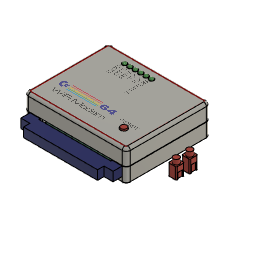
C64-WiFi_UP_PCB2 v9 (Autodesk Fusion 360 design; units mm, degrees)
Autodesk Fusion 360 part; units mm, degrees
note: some values were not read from the file. Set by a fixed rule: which sketch regions a step uses.
(part 1 of 3)
sketch "dxf_import" plane through (0, 0, 0) normal (0, 0, 1) x (1, 0, 0) in component "PCB"
  arc A0 (1, 59) -> (0, 58.08) centre (0.96, 58.04) ccw
  arc A1 (52.3, 0) -> (53.3, 1) centre (52.3, 1) ccw
  arc A2 (53.3, 58.08) -> (52.3, 59) centre (52.34, 58.04) ccw
  circle A3 centre (49.3, 54.7) radius 1.651
  circle A4 centre (4, 12.8) radius 1.651
  line L0 (1, 0) -> (52.3, 0)
  arc A5 (0, 1) -> (1, 0) centre (1, 1) ccw
  arc A6 (48.0347, 39.7544) -> (48.935, 40.0818) centre (48.0347, 41.156) ccw
  line L1 (17.0663, 30.1863) -> (17.0663, 28.2813)
  line L2 (18.6538, 30.8362) -> (19.9238, 31.4713)
  line L3 (21.5113, 30.1863) -> (17.0663, 30.1863)
  line L4 (18.6538, 32.1063) -> (18.6538, 30.8362)
  line L5 (21.543, 34.5271) -> (21.543, 32.6729)
  line L6 (34.0519, 18.9119) -> (34.0519, 17.9594)
  line L7 (33.7344, 18.4944) -> (34.0519, 18.9119)
  line L8 (33.2582, 18.4944) -> (33.2582, 16.2717)
  line L9 (33.0407, 18.9118) -> (33.2582, 18.4944)
  line L10 (21.543, 26.1804) -> (17.987, 26.1804)
  line L11 (33.7345, 16.2718) -> (34.0519, 15.9544)
  line L12 (21.5113, 28.2813) -> (21.5113, 30.1863)
  line L13 (34.0519, 18.9119) -> (32.7819, 18.9119)
  line L14 (17.987, 28.0346) -> (21.543, 28.0346)
  line L15 (17.0663, 32.4237) -> (17.0663, 30.5188)
  line L16 (21.543, 32.6729) -> (17.987, 32.6729)
  line L17 (19.9238, 29.2338) -> (18.6538, 29.8688)
  line L18 (32.7819, 15.8543) -> (33.02, 15.8543)
  line L19 (34.0519, 16.8068) -> (34.0519, 15.9544)
  line L20 (12.4583, 32.4763) -> (12.8392, 32.4763)
  line L21 (9.9183, 28.6663) -> (10.2993, 28.6663)
  line L22 (16.2683, 28.6663) -> (16.3317, 28.6663)
  line L23 (5.5629, 30.3808) -> (7.4171, 30.3808)
  line L24 (18.6538, 29.8688) -> (18.6538, 28.5988)
  line L25 (12.4583, 28.6663) -> (12.8392, 28.6663)
  line L26 (8.6483, 28.6663) -> (9.0293, 28.6663)
  line L27 (17.987, 34.5271) -> (21.543, 34.5271)
  line L28 (17.0663, 28.2813) -> (21.5113, 28.2813)
  line L29 (19.9238, 32.1063) -> (19.9238, 30.8362)
  line L30 (21.5113, 32.4237) -> (17.0663, 32.4237)
  line L31 (7.429, 12.8) -> (6.921, 12.8)
  line L32 (7.6958, 32.4763) -> (7.6958, 28.6663)
  line L33 (11.1883, 28.6663) -> (11.5693, 28.6663)
  line L34 (13.7283, 28.6663) -> (14.1093, 28.6663)
  line L35 (49.3, 51.779) -> (49.3, 51.271)
  circle A7 centre (49.3, 54.7) radius 3.429
  line L36 (8.6483, 32.4763) -> (9.0293, 32.4763)
  line L37 (17.987, 28.0346) -> (17.987, 26.1804)
  line L38 (17.0663, 30.5188) -> (21.5113, 30.5188)
  line L39 (33.7344, 18.4944) -> (33.7344, 16.9068)
  line L40 (21.543, 28.0346) -> (21.543, 26.1804)
  line L41 (18.6538, 28.5988) -> (19.9238, 29.2338)
  line L42 (4, 16.229) -> (4, 15.721)
  line L43 (1.079, 12.8) -> (0.571, 12.8)
  line L44 (5.5629, 33.9368) -> (7.4171, 33.9368)
  line L45 (21.5113, 30.5188) -> (21.5113, 32.4237)
  line L46 (19.9238, 29.8688) -> (19.9238, 28.5988)
  line L47 (17.987, 34.5271) -> (17.987, 32.6729)
  line L48 (34.052, 15.8543) -> (33.0407, 15.8543)
  line L49 (33.7344, 16.9068) -> (33.7345, 16.2718)
  line L50 (33.2582, 18.4944) -> (33.7344, 18.4944)
  line L51 (19.9238, 31.4713) -> (18.6538, 32.1063)
  line L52 (33.2582, 16.2717) -> (33.0407, 15.8543)
  line L53 (5.5629, 30.3808) -> (5.5629, 33.9368)
  line L54 (34.0519, 15.9544) -> (34.052, 15.8543)
  line L55 (7.4171, 33.9368) -> (7.4171, 30.3808)
  circle A8 centre (8.5085, 29.4155) radius 0.5334
  circle A9 centre (4, 12.8) radius 3.429
  line L56 (11.1883, 32.4763) -> (11.5693, 32.4763)
  line L57 (16.2683, 32.4763) -> (16.3317, 32.4763)
  line L58 (33.7345, 16.2718) -> (33.2581, 16.2718)
  line L59 (52.729, 54.7) -> (52.221, 54.7)
  line L60 (7.6958, 32.4763) -> (7.7593, 32.4763)
  line L61 (13.7283, 32.4763) -> (14.1093, 32.4763)
  line L62 (7.6958, 28.6663) -> (7.7593, 28.6663)
  arc A10 (12.9722, 57.9796) -> (12.7372, 58.0579) centre (12.7372, 57.6663) ccw
  line L63 (10.9757, 57.3269) -> (10.9757, 57.8491)
  line L64 (16.0124, 57.1181) -> (16.0124, 58.0579)
  arc A11 (7.3924, 57.7968) -> (7.1313, 58.0579) centre (7.1313, 57.7968) ccw
  line L65 (16.992, 57.5097) -> (16.7048, 57.6663)
  line L66 (19.2861, 58.0579) -> (19.8082, 58.0579)
  arc A12 (7.8126, 57.3269) -> (8.0214, 57.1181) centre (8.0214, 57.3269) ccw
  line L67 (19.5472, 57.1181) -> (19.5472, 58.0579)
  line L68 (11.1845, 58.0579) -> (11.3933, 58.0579)
  line L69 (11.9403, 57.1181) -> (11.9403, 58.0579)
  line L70 (23.5196, 57.5358) -> (23.2585, 57.5358)
  line L71 (8.8687, 57.1181) -> (8.6076, 57.1181)
  line L72 (6.8703, 58.0579) -> (7.1313, 58.0579)
  arc A13 (25.5748, 57.2486) -> (25.8881, 57.1181) centre (25.8881, 57.5593) ccw
  arc A14 (25.601, 57.8491) -> (25.7054, 57.6664) centre (25.8131, 57.8491) ccw
  line L73 (25.9926, 57.5097) -> (25.7054, 57.6663)
  arc A15 (17.0964, 57.3269) -> (16.992, 57.5096) centre (16.8843, 57.3269) ccw
  arc A16 (12.5283, 57.8491) -> (12.6327, 57.6664) centre (12.7404, 57.8491) ccw
  line L74 (15.7513, 58.0579) -> (16.2734, 58.0579)
  line L75 (20.0873, 58.0579) -> (20.7139, 57.1181)
  arc A17 (26.0448, 57.9796) -> (25.8098, 58.0579) centre (25.8098, 57.6663) ccw
  line L76 (14.9036, 57.1181) -> (14.9036, 58.0579)
  arc A18 (12.7372, 58.0579) -> (12.5284, 57.8491) centre (12.7372, 57.8491) ccw
  arc A19 (16.8092, 58.0579) -> (16.6004, 57.8491) centre (16.8092, 57.8491) ccw
  line L77 (15.1647, 57.5358) -> (14.9036, 57.5358)
  line L78 (6.8703, 57.1181) -> (6.8703, 58.0579)
  line L79 (7.8126, 57.3269) -> (7.8126, 57.8491)
  arc A20 (23.5196, 57.5357) -> (23.5196, 58.0579) centre (23.5196, 57.7968) ccw
  line L80 (8.6076, 58.0579) -> (8.8687, 58.0579)
  arc A21 (25.8881, 57.1181) -> (26.0969, 57.3269) centre (25.8881, 57.3269) ccw
  arc A22 (12.8155, 57.1181) -> (13.0243, 57.3269) centre (12.8155, 57.3269) ccw
  line L81 (8.0214, 58.0579) -> (8.2303, 58.0579)
  line L82 (15.4257, 57.1181) -> (15.2169, 57.5358)
  arc A23 (26.097, 57.3269) -> (25.9926, 57.5096) centre (25.8849, 57.3269) ccw
  arc A24 (16.8876, 57.1181) -> (17.0964, 57.3269) centre (16.8876, 57.3269) ccw
  line L83 (23.2585, 58.0579) -> (23.5196, 58.0579)
  arc A25 (16.6004, 57.8491) -> (16.7048, 57.6664) centre (16.8125, 57.8491) ccw
  line L84 (7.1313, 57.1181) -> (6.8703, 57.1181)
  arc A26 (13.0243, 57.3269) -> (12.9199, 57.5096) centre (12.8122, 57.3269) ccw
  line L85 (8.6076, 57.1181) -> (8.6076, 58.0579)
  line L86 (23.2585, 57.1181) -> (23.2585, 58.0579)
  arc A27 (10.9757, 57.3269) -> (11.1845, 57.1181) centre (11.1845, 57.3269) ccw
  line L87 (11.6793, 58.0579) -> (12.2014, 58.0579)
  arc A28 (8.8687, 57.1181) -> (9.1298, 57.3792) centre (8.8687, 57.3792) ccw
  line L88 (14.9036, 58.0579) -> (15.1647, 58.0579)
  arc A29 (7.1313, 57.1181) -> (7.3924, 57.3792) centre (7.1313, 57.3792) ccw
  arc A30 (8.0214, 58.0579) -> (7.8126, 57.8491) centre (8.0214, 57.8491) ccw
  arc A31 (17.0442, 57.9796) -> (16.8092, 58.0579) centre (16.8092, 57.6663) ccw
  line L89 (9.1297, 57.7968) -> (9.1297, 57.3792)
  arc A32 (25.8098, 58.0579) -> (25.601, 57.8491) centre (25.8098, 57.8491) ccw
  line L90 (24.115, 58.0579) -> (24.7415, 57.1181)
  line L91 (27.5123, 58.0579) -> (27.8256, 57.1181)
  arc A33 (11.1845, 58.0579) -> (10.9757, 57.8491) centre (11.1845, 57.8491) ccw
  arc A34 (9.1298, 57.7968) -> (8.8687, 58.0579) centre (8.8687, 57.7968) ccw
  line L92 (23.7806, 57.1181) -> (23.5718, 57.5358)
  line L93 (24.115, 57.1181) -> (24.7415, 58.0579)
  line L94 (28.9886, 58.0579) -> (28.9886, 57.3792)
  arc A35 (12.5022, 57.2486) -> (12.8155, 57.1181) centre (12.8155, 57.5593) ccw
  arc A36 (15.1647, 57.5357) -> (15.1647, 58.0579) centre (15.1647, 57.7968) ccw
  line L95 (8.2303, 57.1181) -> (8.0214, 57.1181)
  line L96 (7.3924, 57.7968) -> (7.3924, 57.3792)
  arc A37 (16.5743, 57.2486) -> (16.8876, 57.1181) centre (16.8876, 57.5593) ccw
  line L97 (28.1047, 58.0579) -> (28.6268, 58.0579)
  line L98 (12.9199, 57.5097) -> (12.6328, 57.6663)
  arc A38 (29.9291, 57.8491) -> (30.0335, 57.6664) centre (30.1412, 57.8491) ccw
  line L99 (26.6589, 57.1181) -> (26.6589, 58.0579)
  line L100 (20.0873, 57.1181) -> (20.7139, 58.0579)
  line L101 (11.3933, 57.1181) -> (11.1845, 57.1181)
  arc A39 (30.2163, 57.1181) -> (30.4251, 57.3269) centre (30.2163, 57.3269) ccw
  line L102 (26.3978, 58.0579) -> (26.9199, 58.0579)
  line L103 (30.3207, 57.5097) -> (30.0335, 57.6663)
  arc A40 (30.4251, 57.3269) -> (30.3207, 57.5096) centre (30.213, 57.3269) ccw
  line L104 (27.7473, 57.3531) -> (27.2774, 57.3531)
  arc A41 (29.903, 57.2486) -> (30.2163, 57.1181) centre (30.2163, 57.5593) ccw
  arc A42 (30.373, 57.9796) -> (30.138, 58.0579) centre (30.138, 57.6663) ccw
  arc A43 (30.138, 58.0579) -> (29.9292, 57.8491) centre (30.138, 57.8491) ccw
  line L105 (28.3658, 57.1181) -> (28.3658, 58.0579)
  line L106 (29.5107, 57.3792) -> (29.5107, 58.0579)
  line L107 (27.1991, 57.1181) -> (27.5123, 58.0579)
  arc A44 (28.9886, 57.3792) -> (29.5108, 57.3792) centre (29.2497, 57.3792) ccw
  arc A45 (48.935, 43.7095) -> (48.0347, 44.0369) centre (48.0347, 42.6353) ccw
  line L108 (16.3317, 28.6663) -> (16.3317, 32.4763)
  line L109 (14.9983, 32.4763) -> (15.3793, 32.4763)
  line L110 (46.379, 54.7) -> (45.871, 54.7)
  line L111 (49.3, 58.129) -> (49.3, 57.621)
  line L112 (4, 9.879) -> (4, 9.371)
  line L113 (14.9983, 28.6663) -> (15.3793, 28.6663)
  line L114 (32.7819, 17.7593) -> (32.7819, 17.0069)
  line L115 (9.9183, 32.4763) -> (10.2993, 32.4763)
  line L116 (34.84, 0) -> (34.34, 0)
  line L117 (34.84, -1) -> (34.84, 0)
  line L118 (49.45, 0.1) -> (49.45, -1)
  line L119 (47.45, 0.1) -> (47.45, -1)
  line L120 (43.49, 0.1) -> (43.49, -1)
  line L121 (37.57, 0.1) -> (37.57, -1)
  line L122 (50.68, -1) -> (50.68, 0)
  line L123 (42.76, -1) -> (42.76, 0)
  line L124 (41.53, 0.1) -> (41.53, -1)
  line L125 (50.68, 0) -> (50.18, 0)
  line L126 (42.26, 0) -> (42.26, -1)
  line L127 (46.72, 0) -> (46.22, 0)
  line L128 (46.22, 0) -> (46.22, -1)
  line L129 (34.34, 0) -> (34.34, -1)
  line L130 (21.73, 0.1) -> (21.73, -1)
  line L131 (26.42, 0) -> (26.42, -1)
  line L132 (38.8, -1) -> (38.8, 0)
  line L133 (39.53, 0.1) -> (39.53, -1)
  line L134 (15.77, 0.1) -> (15.77, -1)
  line L135 (30.38, 0) -> (30.38, -1)
  line L136 (14.54, 0) -> (14.54, -1)
  line L137 (30.88, 0) -> (30.38, 0)
  line L138 (38.8, 0) -> (38.3, 0)
  line L139 (45.49, 0.1) -> (45.49, -1)
  line L140 (35.57, 0.1) -> (35.57, -1)
  line L141 (26.92, 0) -> (26.42, 0)
  line L142 (46.72, -1) -> (46.72, 0)
  line L143 (18.5, 0) -> (18.5, -1)
  line L144 (50.18, 0) -> (50.18, -1)
  line L145 (38.3, 0) -> (38.3, -1)
  line L146 (42.76, 0) -> (42.26, 0)
  line L147 (57.67, -3.6853) -> (57.67, -3.548)
  line L148 (22.46, 0) -> (22.46, -1)
  line L149 (59.37, -6.8) -> (55.97, -6.8)
  line L150 (-6.03, -6.8) -> (-6.03, -5.2)
  line L151 (19.73, 0.1) -> (19.73, -1)
  line L152 (6.62, 0) -> (6.62, -1)
  line L153 (54.17, -6.8) -> (54.17, -11.6)
  line L154 (23.69, 0.1) -> (23.69, -1)
  line L155 (3.89, 0.1) -> (3.89, -1)
  line L156 (57.67, -11.6) -> (57.67, -8.7333)
  line L157 (-6.03, -4.2) -> (-6.03, -2.6)
  line L158 (22.96, 0) -> (22.46, 0)
  line L159 (54.17, -11.6) -> (-0.83, -11.6)
  line L160 (-6.03, -1.6) -> (-6.03, 0)
  line L161 (13.81, 0.1) -> (13.81, -1)
  line L162 (11.81, 0.1) -> (11.81, -1)
  line L163 (30.88, -1) -> (30.88, 0)
  line L164 (17.77, 0.1) -> (17.77, -1)
  line L165 (10.58, 0) -> (10.58, -1)
  line L166 (57.67, -8.052) -> (57.67, -7.9147)
  line L167 (-0.13, -1) -> (-0.13, 0)
  line L168 (5.89, 0.1) -> (5.89, -1)
  line L169 (25.69, 0.1) -> (25.69, -1)
  line L170 (19, -1) -> (19, 0)
  line L171 (11.08, 0) -> (10.58, 0)
  line L172 (26.92, -1) -> (26.92, 0)
  line L173 (29.65, 0.1) -> (29.65, -1)
  line L174 (31.61, 0.1) -> (31.61, -1)
  line L175 (11.08, -1) -> (11.08, 0)
  line L176 (15.04, 0) -> (14.54, 0)
  line L177 (27.65, 0.1) -> (27.65, -1)
  line L178 (9.85, 0.1) -> (9.85, -1)
  line L179 (-2.63, -6.8) -> (-6.03, -6.8)
  line L180 (19, 0) -> (18.5, 0)
  line L181 (60.92, 0) -> (59.37, 0)
  line L182 (-4.33, -3.548) -> (-4.33, -3.6853)
  line L183 (33.61, 0.1) -> (33.61, -1)
  line L184 (-4.33, -4.3667) -> (-4.33, -7.2333)
  line L185 (22.96, -1) -> (22.96, 0)
  line L186 (15.04, -1) -> (15.04, 0)
  line L187 (7.12, 0) -> (6.62, 0)
  line L188 (-0.13, 0) -> (-2.63, 0)
  line L189 (12.1444, 18.9706) -> (13.4144, 18.9706)
  line L190 (31.8294, 18.3356) -> (31.8294, 17.0656)
  line L191 (16.5894, 18.3356) -> (17.2244, 18.9706)
  line L192 (29.9244, 18.9706) -> (29.2894, 18.3356)
  line L193 (7.12, -1) -> (7.12, 0)
  line L194 (59.37, -1.6) -> (59.37, 0)
  line L195 (31.8294, 17.0656) -> (31.1944, 16.4306)
  line L196 (26.1144, 16.4306) -> (24.8444, 16.4306)
  line L197 (26.1144, 18.9706) -> (26.7494, 18.3356)
  line L198 (55.97, -6.8) -> (55.97, -5.2)
  line L199 (19.7644, 18.9706) -> (21.0344, 18.9706)
  line L200 (19.1294, 17.0656) -> (18.4944, 16.4306)
  line L201 (55.97, -1.6) -> (55.97, 0)
  line L202 (-2.63, 0) -> (-4.33, 0)
  line L203 (29.2894, 18.3356) -> (29.2894, 17.0656)
  line L204 (24.2094, 18.3356) -> (24.8444, 18.9706)
  line L205 (21.0344, 16.4306) -> (19.7644, 16.4306)
  line L206 (7.85, 0.1) -> (7.85, -1)
  line L207 (-4.33, -7.9147) -> (-4.33, -8.052)
  line L208 (-2.63, -6.8) -> (-2.63, -5.2)
  line L209 (-4.33, 0) -> (-4.33, -2.8667)
  line L210 (26.7494, 17.0656) -> (27.3844, 16.4306)
  line L211 (-6.03, 0) -> (-7.58, 0)
  line L212 (59.37, -4.2) -> (59.37, -2.6)
  line L213 (12.1444, 18.9706) -> (11.5094, 18.3356)
  line L214 (60.92, -6.8) -> (59.37, -6.8)
  line L215 (26.7494, 18.3356) -> (26.7494, 17.0656)
  line L216 (-2.63, -4.2) -> (-2.63, -2.6)
  line L217 (55.97, 0) -> (53.47, 0)
  line L218 (60.92, 0) -> (60.92, -6.8)
  line L219 (53.47, 0) -> (53.47, -1)
  line L220 (57.67, 0) -> (55.97, 0)
  line L221 (3.16, 0) -> (2.66, 0)
  line L222 (-4.33, 0) -> (-6.03, 0)
  line L223 (2.66, 0) -> (2.66, -1)
  line L224 (-0.83, -6.8) -> (-2.63, -6.8)
  line L225 (24.2094, 17.0656) -> (23.5744, 16.4306)
  line L226 (21.6694, 18.3356) -> (21.6694, 17.0656)
  line L227 (14.0494, 18.3356) -> (14.0494, 17.0656)
  line L228 (29.2894, 17.0656) -> (28.6544, 16.4306)
  line L229 (15.9544, 18.9706) -> (16.5894, 18.3356)
  line L230 (21.6694, 18.3356) -> (22.3044, 18.9706)
  line L231 (24.8444, 16.4306) -> (24.2094, 17.0656)
  line L232 (13.4144, 16.4306) -> (12.1444, 16.4306)
  line L233 (28.6544, 16.4306) -> (27.3844, 16.4306)
  line L234 (59.37, 0) -> (57.67, 0)
  line L235 (14.0494, 18.3356) -> (14.6844, 18.9706)
  line L236 (55.97, -6.8) -> (54.17, -6.8)
  line L237 (57.67, -2.8667) -> (57.67, 0)
  line L238 (3.16, -1) -> (3.16, 0)
  line L239 (-0.83, -11.6) -> (-0.83, -6.8)
  line L240 (-6.03, -6.8) -> (-7.58, -6.8)
  line L241 (53.47, -1) -> (-0.13, -1)
  line L242 (57.67, -7.2333) -> (57.67, -4.3667)
  line L243 (18.4944, 16.4306) -> (17.2244, 16.4306)
  line L244 (13.4144, 18.9706) -> (14.0494, 18.3356)
  line L245 (11.5094, 18.3356) -> (11.5094, 17.0656)
  line L246 (-4.33, -8.7333) -> (-4.33, -11.6)
  line L247 (17.2244, 16.4306) -> (16.5894, 17.0656)
  line L248 (27.3844, 18.9706) -> (28.6544, 18.9706)
  line L249 (59.37, -6.8) -> (59.37, -5.2)
  line L250 (-7.58, 0) -> (-7.58, -6.8)
  line L251 (19.1294, 18.3356) -> (19.1294, 17.0656)
  line L252 (14.6844, 16.4306) -> (14.0494, 17.0656)
  line L253 (6.8887, 53.0538) -> (6.2538, 53.0538)
  line L254 (18.8888, 53.0538) -> (18.2538, 53.0538)
  arc A46 (24.8, 53.2) -> (24.8, 56.2) centre (24, 54.7) ccw
  line L255 (14.5713, 53.3713) -> (14.5713, 52.7363)
  line L256 (16.5894, 17.0656) -> (15.9544, 16.4306)
  line L257 (14.0494, 17.0656) -> (13.4144, 16.4306)
  arc A47 (20.8, 53.2) -> (20.8, 56.2) centre (20, 54.7) ccw
  line L258 (19.7644, 18.9706) -> (19.1294, 18.3356)
  line L259 (22.3044, 18.9706) -> (23.5744, 18.9706)
  line L260 (10.8887, 53.0538) -> (10.2538, 53.0538)
  arc A48 (23.2, 56.2) -> (23.2, 53.2) centre (24, 54.7) ccw
  line L261 (18.8888, 56.2875) -> (18.2538, 56.2875)
  arc A49 (19.2, 56.2) -> (19.2, 53.2) centre (20, 54.7) ccw
  arc A50 (8.8, 53.2) -> (8.8, 56.2) centre (8, 54.7) ccw
  arc A51 (24.8, 53.2) -> (24.8, 56.2) centre (24, 54.7) ccw
  line L262 (22.5713, 53.3713) -> (22.5713, 52.7363)
  arc A52 (23.2, 56.2) -> (23.2, 53.2) centre (24, 54.7) ccw
  line L263 (22.8888, 56.2875) -> (22.2538, 56.2875)
  line L264 (22.8888, 53.0538) -> (22.2538, 53.0538)
  arc A53 (7.2, 56.2) -> (7.2, 53.2) centre (8, 54.7) ccw
  arc A54 (12.8, 53.2) -> (12.8, 56.2) centre (12, 54.7) ccw
  arc A55 (15.2, 56.2) -> (15.2, 53.2) centre (16, 54.7) ccw
  arc A56 (20.8, 53.2) -> (20.8, 56.2) centre (20, 54.7) ccw
  arc A57 (7.2, 56.2) -> (7.2, 53.2) centre (8, 54.7) ccw
  line L265 (18.5712, 53.3713) -> (18.5712, 52.7363)
  arc A58 (16.8, 53.2) -> (16.8, 56.2) centre (16, 54.7) ccw
  line L266 (6.8887, 56.2875) -> (6.2538, 56.2875)
  line L267 (55.97, -4.2) -> (55.97, -2.6)
  line L268 (27.3844, 18.9706) -> (26.7494, 18.3356)
  line L269 (21.6694, 17.0656) -> (21.0344, 16.4306)
  line L270 (14.6844, 18.9706) -> (15.9544, 18.9706)
  line L271 (23.5744, 18.9706) -> (24.2094, 18.3356)
  line L272 (22.3044, 16.4306) -> (21.6694, 17.0656)
  line L273 (16.5894, 18.3356) -> (16.5894, 17.0656)
  line L274 (-2.63, -1.6) -> (-2.63, 0)
  line L275 (21.0344, 18.9706) -> (21.6694, 18.3356)
  line L276 (24.2094, 18.3356) -> (24.2094, 17.0656)
  line L277 (10.8887, 56.2875) -> (10.2538, 56.2875)
  line L278 (29.9244, 18.9706) -> (31.1944, 18.9706)
  line L279 (28.6544, 18.9706) -> (29.2894, 18.3356)
  line L280 (31.1944, 18.9706) -> (31.8294, 18.3356)
  line L281 (31.1944, 16.4306) -> (29.9244, 16.4306)
  line L282 (11.5094, 16.4306) -> (12.1444, 16.4306)
  arc A59 (11.2, 56.2) -> (11.2, 53.2) centre (12, 54.7) ccw
  line L283 (11.5094, 17.0656) -> (11.5094, 16.4306)
  line L284 (29.2894, 17.0656) -> (29.9244, 16.4306)
  arc A60 (15.2, 56.2) -> (15.2, 53.2) centre (16, 54.7) ccw
  line L285 (14.8887, 53.0538) -> (14.2538, 53.0538)
  line L286 (26.7494, 17.0656) -> (26.1144, 16.4306)
  line L287 (6.5713, 53.3713) -> (6.5713, 52.7363)
  line L288 (14.8887, 56.2875) -> (14.2538, 56.2875)
  line L289 (10.5713, 53.3713) -> (10.5713, 52.7363)
  line L290 (18.4944, 18.9706) -> (19.1294, 18.3356)
  arc A61 (16.8, 53.2) -> (16.8, 56.2) centre (16, 54.7) ccw
  line L291 (17.2244, 18.9706) -> (18.4944, 18.9706)
  arc A62 (19.2, 56.2) -> (19.2, 53.2) centre (20, 54.7) ccw
  line L292 (24.8444, 18.9706) -> (26.1144, 18.9706)
  arc A63 (12.8, 53.2) -> (12.8, 56.2) centre (12, 54.7) ccw
  line L293 (15.9544, 16.4306) -> (14.6844, 16.4306)
  line L294 (23.5744, 16.4306) -> (22.3044, 16.4306)
  line L295 (19.1294, 17.0656) -> (19.7644, 16.4306)
  arc A64 (11.2, 56.2) -> (11.2, 53.2) centre (12, 54.7) ccw
  arc A65 (8.8, 53.2) -> (8.8, 56.2) centre (8, 54.7) ccw
  line L296 (49.1, 37.695) -> (49.1, 38.7138)
  line L297 (49.1, 39.7138) -> (49.1, 40.7325)
  line L298 (45.0724, 50.8263) -> (44.0586, 50.8263)
  line L299 (28.9621, 50.8263) -> (27.9483, 50.8263)
  line L300 (40.4, 39.7263) -> (40.4, 38.9263)
  line L301 (44.4, 36.9263) -> (44.4, 39.7263)
  line L302 (20.9069, 50.8263) -> (19.8931, 50.8263)
  line L303 (10.8379, 50.8263) -> (9.8241, 50.8263)
  line L304 (-8.3, 23.5638) -> (-8.3, 24.5825)
  line L305 (-8.3, 39.7138) -> (-8.3, 40.7325)
  line L306 (40.4, 27.2263) -> (40.4, 24.4262)
  line L307 (40.5, 36.0263) -> (45.8, 36.0263)
  line L308 (44.8, 31.5263) -> (44.8, 39.2263)
  line L309 (-8.3, 43.7512) -> (-8.3, 44.77)
  line L310 (44.53, 44.9263) -> (44.5, 44.9263)
  line L311 (44.4, 24.4262) -> (44.4, 27.2263)
  line L312 (49.1, 25.5825) -> (49.1, 26.6013)
  line L313 (40.4, 24.4262) -> (44.4, 24.4262)
  line L314 (8.8241, 50.8263) -> (7.8103, 50.8263)
  line L315 (49.1, 31.6388) -> (49.1, 32.6575)
  line L316 (49.1, 47.7888) -> (49.1, 48.8075)
  line L317 (26.9483, 50.8263) -> (25.9345, 50.8263)
  line L318 (44.5, 44.9263) -> (-3.7, 44.9263)
  line L319 (44.4, 39.7263) -> (40.4, 39.7263)
  line L320 (-3.7, 44.9263) -> (-3.73, 44.9263)
  line L321 (40.4, 28.3263) -> (40.4, 36.0263)
  arc A66 (27.2, 56.2) -> (27.2, 53.2) centre (28, 54.7) ccw
  line L322 (40.4, 38.9263) -> (40.4, 36.9263)
  arc A67 (28.8, 53.2) -> (28.8, 56.2) centre (28, 54.7) ccw
  line L323 (40.4, 36.9263) -> (44.4, 36.9263)
  arc A68 (28.8, 53.2) -> (28.8, 56.2) centre (28, 54.7) ccw
  line L324 (26.5713, 53.3713) -> (26.5713, 52.7363)
  line L325 (26.8888, 56.2875) -> (26.2538, 56.2875)
  line L326 (40.4, 36.0263) -> (40.5, 36.0263)
  line L327 (44.4, 27.2263) -> (40.4, 27.2263)
  line L328 (12.8517, 50.8263) -> (11.8379, 50.8263)
  line L329 (-8.3, 41.7325) -> (-8.3, 42.7512)
  line L330 (44.8, 19.5263) -> (-4, 19.5263)
  line L331 (-8.3, 21.545) -> (-8.3, 22.5638)
  line L332 (49.1, 21.545) -> (49.1, 22.5638)
  line L333 (49.1, 27.6013) -> (49.1, 28.62)
  line L334 (-8.3, 31.6388) -> (-8.3, 32.6575)
  line L335 (26.8888, 53.0538) -> (26.2538, 53.0538)
  arc A69 (27.2, 56.2) -> (27.2, 53.2) centre (28, 54.7) ccw
  line L336 (45.8, 28.3263) -> (40.4, 28.3263)
  line L337 (40.4, 36.0263) -> (40.5, 36.0263)
  line L338 (45.8, 36.0263) -> (45.8, 28.3263)
  line L339 (-4, 19.5263) -> (-5.65, 19.5263)
  line L340 (30.9759, 50.8263) -> (29.9621, 50.8263)
  line L341 (37.0172, 50.8263) -> (36.0034, 50.8263)
  line L342 (50.1, 31.5263) -> (49, 31.5263)
  line L343 (45.9, 31.5263) -> (44.8, 31.5263)
  line L344 (-8.3, 33.6575) -> (-8.3, 34.6763)
  line L345 (-8.3, 35.6763) -> (-8.3, 36.695)
  line L346 (-8.3, 47.7888) -> (-8.3, 48.8075)
  line L347 (24.9345, 50.8263) -> (23.9207, 50.8263)
  line L348 (-8.3, 29.62) -> (-8.3, 30.6388)
  line L349 (44.8, 19.5263) -> (44.8, 31.5263)
  line L350 (-8.3, 37.695) -> (-8.3, 38.7138)
  line L351 (16.8793, 50.8263) -> (15.8655, 50.8263)
  line L352 (44.8, 39.2263) -> (44.8, 44.9263)
  line L353 (49.1, 49.8075) -> (49.1, 50.8263)
  line L354 (43.0586, 50.8263) -> (42.0448, 50.8263)
  line L355 (-8.3, 25.5825) -> (-8.3, 26.6013)
  line L356 (44.8, 19.5263) -> (46.45, 19.5263)
  line L357 (49.1, 19.5263) -> (49.1, 20.545)
  line L358 (49.1, 41.7325) -> (49.1, 42.7512)
  line L359 (41.0448, 50.8263) -> (40.031, 50.8263)
  line L360 (-8.3, 27.6013) -> (-8.3, 28.62)
  line L361 (-6.65, 19.5263) -> (-8.3, 19.5263)
  line L362 (49.1, 43.7512) -> (49.1, 44.77)
  line L363 (6.8103, 50.8263) -> (5.7966, 50.8263)
  line L364 (49.1, 45.77) -> (49.1, 46.7888)
  line L365 (49.1, 29.62) -> (49.1, 30.6388)
  line L366 (49.1, 33.6575) -> (49.1, 34.6763)
  line L367 (47.45, 19.5263) -> (49.1, 19.5263)
  line L368 (22.9207, 50.8263) -> (21.9069, 50.8263)
  line L369 (-8.3, 45.77) -> (-8.3, 46.7888)
  line L370 (49.1, 23.5638) -> (49.1, 24.5825)
  line L371 (14.8655, 50.8263) -> (13.8517, 50.8263)
  line L372 (47.0862, 50.8263) -> (46.0724, 50.8263)
  line L373 (39.031, 50.8263) -> (38.0172, 50.8263)
  line L374 (49.1, 35.6763) -> (49.1, 36.695)
  line L375 (49.1, 50.8263) -> (48.0862, 50.8263)
  line L376 (-4, 19.5263) -> (-4, 44.9263)
  line L377 (32.9897, 50.8263) -> (31.9759, 50.8263)
  line L378 (18.8931, 50.8263) -> (17.8793, 50.8263)
  line L379 (-4, 44.9263) -> (-3.7, 44.9263)
  line L380 (2.7828, 50.8263) -> (1.769, 50.8263)
  line L381 (44.8, 44.9263) -> (44.5, 44.9263)
  line L382 (35.0034, 50.8263) -> (33.9897, 50.8263)
  line L383 (-8.3, 49.8075) -> (-8.3, 50.8263)
  line L384 (-8.3, 19.5263) -> (-8.3, 20.545)
  line L385 (44.8, 39.2263) -> (45.9, 39.2263)
  line L386 (50.1, 34.8762) -> (50.1, 33.7013)
  line L387 (49, 39.2263) -> (50.1, 39.2263)
  line L388 (4.7966, 50.8263) -> (3.7828, 50.8263)
  line L389 (-1.2448, 50.8263) -> (-2.2586, 50.8263)
  line L390 (0.769, 50.8263) -> (-0.2448, 50.8263)
  line L391 (50.1, 37.0513) -> (50.1, 35.8762)
  line L392 (50.1, 32.7013) -> (50.1, 31.5263)
  line L393 (50.1, 39.2263) -> (50.1, 38.0513)
  line L394 (-7.2862, 50.8263) -> (-8.3, 50.8263)
  line L395 (-3.2586, 50.8263) -> (-4.2724, 50.8263)
  line L396 (-5.2724, 50.8263) -> (-6.2862, 50.8263)
  line L397 (35.4012, 10.4774) -> (35.4012, 10.9538)
  line L398 (14.7275, 11.43) -> (14.7275, 11.1919)
  line L399 (38.0413, 10.16) -> (37.0888, 10.16)
  line L400 (35.0838, 10.16) -> (34.9837, 10.1599)
  line L401 (14.8276, 10.16) -> (14.7275, 10.1599)
  circle A70 centre (42.4, 25.8263) radius 0.9
  line L402 (35.4011, 10.9537) -> (34.9837, 11.1712)
  line L403 (38.0412, 11.1712) -> (37.6238, 10.9537)
  line L404 (38.0413, 10.16) -> (38.0413, 11.43)
  line L405 (17.3676, 10.9537) -> (15.1448, 10.9537)
  line L406 (14.7275, 10.1599) -> (14.7275, 11.1712)
  line L407 (36.0362, 10.4775) -> (35.4012, 10.4774)
  line L408 (17.3676, 10.9537) -> (17.3676, 10.4775)
  line L409 (15.145, 10.4774) -> (14.8276, 10.16)
  line L410 (37.6238, 10.4775) -> (38.0413, 10.16)
  line L411 (35.9362, 10.16) -> (35.0838, 10.16)
  line L412 (15.78, 10.4775) -> (15.145, 10.4774)
  line L413 (17.7851, 10.16) -> (16.8326, 10.16)
  line L414 (15.68, 10.16) -> (14.8276, 10.16)
  line L415 (17.7851, 10.16) -> (17.7851, 11.43)
  line L416 (28.6551, 34.5226) -> (28.6551, 34.0462)
  line L417 (26.4325, 34.0463) -> (26.4325, 34.5225)
  line L418 (37.6238, 10.4775) -> (36.0362, 10.4775)
  line L419 (17.3676, 10.4775) -> (15.78, 10.4775)
  line L420 (24.665, 10.16) -> (23.8126, 10.16)
  line L421 (32.385, 10.4775) -> (32.8026, 10.16)
  line L422 (26.4325, 34.5225) -> (26.015, 34.84)
  line L423 (30.7975, 10.4775) -> (30.1624, 10.4774)
  line L424 (32.8026, 10.16) -> (31.8501, 10.16)
  line L425 (32.8026, 10.16) -> (32.8026, 11.43)
  line L426 (31.65, 11.43) -> (30.8976, 11.43)
  line L427 (37.6238, 10.9537) -> (37.6238, 10.4775)
  line L428 (36.8887, 11.43) -> (36.1363, 11.43)
  line L429 (15.1448, 10.9537) -> (14.7275, 11.1712)
  line L430 (17.785, 11.1712) -> (17.3676, 10.9537)
  line L431 (44.4501, 10.9537) -> (42.2274, 10.9537)
  line L432 (41.81, 10.1599) -> (41.81, 11.1712)
  line L433 (42.8625, 10.4775) -> (42.2275, 10.4774)
  line L434 (42.2275, 10.4774) -> (41.9101, 10.16)
  line L435 (41.81, 11.43) -> (41.81, 11.1919)
  line L436 (26.4325, 34.5225) -> (28.0201, 34.5225)
  line L437 (44.8675, 11.1712) -> (44.4501, 10.9537)
  line L438 (44.4501, 10.9537) -> (44.4501, 10.4775)
  line L439 (23.8126, 10.16) -> (23.7125, 10.1599)
  line L440 (44.8676, 10.16) -> (43.9151, 10.16)
  line L441 (26.0151, 33.8288) -> (26.4325, 34.0463)
  line L442 (35.4012, 10.4774) -> (35.0838, 10.16)
  line L443 (16.6325, 11.43) -> (15.8801, 11.43)
  line L444 (32.385, 10.9537) -> (30.1623, 10.9537)
  line L445 (23.7125, 11.43) -> (23.7125, 11.1919)
  line L446 (26.7701, 10.16) -> (26.7701, 11.43)
  line L447 (29.8451, 10.16) -> (29.745, 10.1599)
  line L448 (26.3526, 10.9537) -> (24.1299, 10.9537)
  line L449 (26.3526, 10.4775) -> (24.765, 10.4775)
  line L450 (34.9837, 10.1599) -> (34.9837, 11.1712)
  line L451 (17.3676, 10.4775) -> (17.7851, 10.16)
  line L452 (37.6238, 10.9537) -> (35.4011, 10.9537)
  circle A71 centre (42.4, 38.3263) radius 0.9
  line L453 (23.7125, 10.1599) -> (23.7125, 11.1712)
  line L454 (30.1623, 10.9537) -> (29.745, 11.1712)
  line L455 (15.145, 10.4774) -> (15.145, 10.9538)
  line L456 (26.3526, 10.4775) -> (26.7701, 10.16)
  line L457 (24.13, 10.4774) -> (23.8126, 10.16)
  line L458 (34.9837, 11.43) -> (34.9837, 11.1919)
  line L459 (32.385, 10.4775) -> (30.7975, 10.4775)
  line L460 (32.385, 10.9537) -> (32.385, 10.4775)
  line L461 (26.7701, 10.16) -> (25.8176, 10.16)
  line L462 (30.1624, 10.4774) -> (29.8451, 10.16)
  line L463 (32.8025, 11.1712) -> (32.385, 10.9537)
  line L464 (30.6974, 10.16) -> (29.8451, 10.16)
  line L465 (24.765, 10.4775) -> (24.13, 10.4774)
  line L466 (25.6175, 11.43) -> (24.8651, 11.43)
  line L467 (30.1624, 10.4774) -> (30.1624, 10.9538)
  line L468 (24.13, 10.4774) -> (24.13, 10.9538)
  line L469 (28.6552, 34.0463) -> (29.0725, 33.8288)
  line L470 (26.77, 11.1712) -> (26.3526, 10.9537)
  line L471 (28.6551, 34.5226) -> (28.9725, 34.84)
  line L472 (24.1299, 10.9537) -> (23.7125, 11.1712)
  line L473 (44.4501, 10.4775) -> (44.8676, 10.16)
  line L474 (26.3526, 10.9537) -> (26.3526, 10.4775)
  line L475 (29.745, 10.1599) -> (29.745, 11.1712)
  line L476 (43.715, 11.43) -> (42.9626, 11.43)
  line L477 (42.2274, 10.9537) -> (41.81, 11.1712)
  line L478 (28.9725, 34.84) -> (29.0725, 34.8401)
  line L479 (25.8562, 28.7288) -> (25.8562, 27.4588)
  line L480 (36.9687, 56.59) -> (37.9212, 56.59)
  line L481 (34.7345, 14.4209) -> (34.7345, 12.5667)
  line L482 (38.2905, 7.3279) -> (38.2905, 9.1821)
  line L483 (27.0192, 7.3279) -> (23.4633, 7.3279)
  line L484 (26.015, 34.84) -> (26.9675, 34.84)
  line L485 (18.193, 14.4209) -> (18.193, 12.5667)
  line L486 (23.4633, 9.1821) -> (27.0192, 9.1821)
  line L487 (26.2737, 27.9351) -> (28.4964, 27.9351)
  line L488 (26.4325, 34.0463) -> (28.6552, 34.0463)
  line L489 (14.637, 9.1821) -> (18.193, 9.1821)
  line L490 (28.4964, 27.9351) -> (28.9138, 27.7176)
  line L491 (28.9138, 27.4588) -> (28.9138, 27.6968)
  line L492 (38.2905, 12.5667) -> (34.7345, 12.5667)
  line L493 (34.7345, 14.4209) -> (38.2905, 14.4209)
  line L494 (33.0517, 7.3279) -> (33.0517, 9.1821)
  line L495 (23.4633, 14.4209) -> (23.4633, 12.5667)
  line L496 (44.4501, 10.4775) -> (42.8625, 10.4775)
  line L497 (37.3862, 56.2725) -> (38.9738, 56.2725)
  line L498 (26.2737, 27.9351) -> (26.2737, 28.4113)
  line L499 (27.0192, 12.5667) -> (23.4633, 12.5667)
  line L500 (37.3862, 55.7963) -> (37.3862, 56.2725)
  line L501 (36.9687, 56.59) -> (36.9687, 55.32)
  line L502 (38.9738, 56.2725) -> (39.6088, 56.2726)
  line L503 (29.745, 11.43) -> (29.745, 11.1919)
  line L504 (29.337, 14.4209) -> (32.893, 14.4209)
  line L505 (18.193, 7.3279) -> (14.637, 7.3279)
  line L506 (32.893, 12.5667) -> (29.337, 12.5667)
  line L507 (41.9101, 10.16) -> (41.81, 10.1599)
  line L508 (27.0088, 27.4588) -> (27.7612, 27.4588)
  line L509 (28.4963, 28.4114) -> (28.8137, 28.7288)
  line L510 (25.8563, 27.7176) -> (26.2737, 27.9351)
  line L511 (18.193, 12.5667) -> (14.637, 12.5667)
  line L512 (42.7625, 10.16) -> (41.9101, 10.16)
  line L513 (39.6089, 55.7963) -> (40.0263, 55.5788)
  line L514 (29.0725, 33.57) -> (29.0725, 33.8081)
  line L515 (44.8676, 10.16) -> (44.8676, 11.43)
  line L516 (29.4958, 7.3279) -> (29.4958, 9.1821)
  line L517 (40.0263, 55.32) -> (40.0263, 55.5581)
  line L518 (34.7345, 7.3279) -> (34.7345, 9.1821)
  line L519 (28.0201, 34.5225) -> (28.6551, 34.5226)
  line L520 (27.1676, 33.57) -> (27.92, 33.57)
  line L521 (36.9688, 55.5788) -> (37.3862, 55.7963)
  line L522 (40.0263, 56.5901) -> (40.0263, 55.5788)
  line L523 (26.015, 34.84) -> (26.015, 33.57)
  line L524 (28.9138, 28.7289) -> (28.9138, 27.7176)
  line L525 (25.8562, 28.7288) -> (26.8087, 28.7288)
  line L526 (27.9613, 28.7288) -> (28.8137, 28.7288)
  line L527 (34.7345, 9.1821) -> (38.2905, 9.1821)
  line L528 (28.8137, 28.7288) -> (28.9138, 28.7289)
  line L529 (26.2737, 28.4113) -> (25.8562, 28.7288)
  line L530 (38.2905, 7.3279) -> (34.7345, 7.3279)
  line L531 (39.6088, 56.2726) -> (39.9262, 56.59)
  line L532 (28.4963, 28.4114) -> (28.4963, 27.935)
  line L533 (37.3862, 56.2725) -> (36.9687, 56.59)
  line L534 (29.4958, 9.1821) -> (33.0517, 9.1821)
  line L535 (38.1213, 55.32) -> (38.8737, 55.32)
  line L536 (42.2275, 10.4774) -> (42.2275, 10.9538)
  line L537 (29.0725, 34.8401) -> (29.0725, 33.8288)
  line L538 (27.8613, 28.4113) -> (28.4963, 28.4114)
  line L539 (28.1201, 34.84) -> (28.9725, 34.84)
  line L540 (26.2737, 28.4113) -> (27.8613, 28.4113)
  line L541 (27.0192, 14.4209) -> (27.0192, 12.5667)
  line L542 (37.3862, 55.7963) -> (39.6089, 55.7963)
  line L543 (29.337, 14.4209) -> (29.337, 12.5667)
  line L544 (25.5118, 28.0671) -> (25.5118, 26.2129)
  line L545 (22.1145, 34.5596) -> (22.1145, 32.7054)
  line L546 (30.8445, 54.8454) -> (30.8445, 56.6996)
  line L547 (25.6705, 32.7054) -> (22.1145, 32.7054)
  line L548 (34.4005, 54.8454) -> (34.4005, 56.6996)
  line L549 (9.7542, 38.053) -> (11.6083, 38.053)
  line L550 (14.2909, 38.053) -> (14.2909, 34.497)
  line L551 (18.193, 7.3279) -> (18.193, 9.1821)
  line L552 (38.5859, 54.2455) -> (38.5859, 50.6895)
  line L553 (14.637, 14.4209) -> (14.637, 12.5667)
  line L554 (44.958, 14.4209) -> (44.958, 12.5667)
  line L555 (34.4005, 50.6629) -> (30.8445, 50.6629)
  line L556 (45.1168, 7.3279) -> (45.1168, 9.1821)
  line L557 (14.9604, 34.497) -> (14.9604, 38.053)
  line L558 (39.6088, 56.2726) -> (39.6088, 55.7962)
  line L559 (33.0517, 7.3279) -> (29.4958, 7.3279)
  line L560 (45.1168, 7.3279) -> (41.5607, 7.3279)
  line L561 (30.8445, 54.5646) -> (34.4005, 54.5646)
  line L562 (30.8445, 56.6996) -> (34.4005, 56.6996)
  line L563 (39.0738, 56.59) -> (39.9262, 56.59)
  line L564 (39.9262, 56.59) -> (40.0263, 56.5901)
  line L565 (34.4005, 54.8454) -> (30.8445, 54.8454)
  line L566 (14.637, 7.3279) -> (14.637, 9.1821)
  line L567 (21.9558, 28.0671) -> (25.5118, 28.0671)
  line L568 (41.5607, 7.3279) -> (41.5607, 9.1821)
  line L569 (30.8445, 52.7104) -> (30.8445, 54.5646)
  line L570 (23.4633, 14.4209) -> (27.0192, 14.4209)
  line L571 (23.4633, 7.3279) -> (23.4633, 9.1821)
  line L572 (46.3, 10.05) -> (46.3, 15.55)
  line L573 (32.893, 14.4209) -> (32.893, 12.5667)
  line L574 (16.8146, 38.053) -> (16.8146, 34.497)
  line L575 (27.0192, 7.3279) -> (27.0192, 9.1821)
  line L576 (25.5118, 26.2129) -> (21.9558, 26.2129)
  line L577 (41.402, 14.4209) -> (44.958, 14.4209)
  line L578 (14.9604, 38.053) -> (16.8146, 38.053)
  line L579 (36.7317, 54.2455) -> (38.5859, 54.2455)
  line L580 (36.7317, 50.6895) -> (36.7317, 54.2455)
  line L581 (38.2905, 14.4209) -> (38.2905, 12.5667)
  line L582 (21.9558, 28.0671) -> (21.9558, 26.2129)
  line L583 (14.9604, 34.497) -> (16.8146, 34.497)
  line L584 (9.7542, 34.497) -> (9.7542, 38.053)
  line L585 (9.7542, 34.497) -> (11.6083, 34.497)
  line L586 (41.5607, 9.1821) -> (45.1168, 9.1821)
  line L587 (12.4367, 34.497) -> (14.2909, 34.497)
  line L588 (14.637, 14.4209) -> (18.193, 14.4209)
  line L589 (34.4005, 50.6629) -> (34.4005, 52.5171)
  line L590 (30.8445, 52.5171) -> (34.4005, 52.5171)
  line L591 (22.1145, 34.5596) -> (25.6705, 34.5596)
  line L592 (12.4367, 34.497) -> (12.4367, 38.053)
  line L593 (44.958, 12.5667) -> (41.402, 12.5667)
  line L594 (41.402, 14.4209) -> (41.402, 12.5667)
  line L595 (34.4005, 52.7104) -> (34.4005, 54.5646)
  line L596 (36.7317, 50.6895) -> (38.5859, 50.6895)
  line L597 (25.6705, 34.5596) -> (25.6705, 32.7054)
  line L598 (34.4005, 52.7104) -> (30.8445, 52.7104)
  line L599 (12.4367, 38.053) -> (14.2909, 38.053)
  line L600 (11.6083, 38.053) -> (11.6083, 34.497)
  line L601 (30.8445, 50.6629) -> (30.8445, 52.5171)
  arc A72 (51.05, 15.25) -> (51.85, 15.25) centre (51.45, 14.95) ccw
  line L602 (52.3, 15.2) -> (52.3, 10.05)
  arc A73 (47.55, 10.35) -> (46.8, 10.3) centre (47.1533, 10.6502) ccw
  line L603 (47.85, 15.8) -> (50.7, 15.8)
  circle A74 centre (49.3, 12.8) radius 1.75
  circle A75 centre (49.3, 12.8) radius 1.4
  arc A76 (46.75, 15.25) -> (47.5, 15.3) centre (47.1467, 14.9498) ccw
  line L604 (50.75, 9.8) -> (47.85, 9.8)
  arc A77 (51.85, 10.35) -> (51.1, 10.3) centre (51.4533, 10.6502) ccw
  arc A78 (46.3, 10) -> (46.5, 9.8) centre (46.5, 10) ccw
  line L605 (46.3, 15.55) -> (46.3, 15.6)
  line L606 (52.3, 15.6) -> (52.3, 15.2)
  line L607 (46.5, 15.8) -> (47.85, 15.8)
  line L608 (26.115, 27.4588) -> (26.75, 27.4588)
  line L609 (27.0675, 28.7288) -> (27.7025, 28.7288)
  line L610 (26.2737, 33.57) -> (26.9088, 33.57)
  line L611 (38.815, 55.32) -> (39.1325, 55.32)
  line L612 (39.7675, 54.685) -> (39.7675, 55.32)
  line L613 (39.1325, 54.685) -> (39.7675, 54.685)
  line L614 (37.2275, 55.32) -> (37.2275, 54.685)
  line L615 (38.815, 56.59) -> (39.1325, 56.59)
  line L616 (51.9, 9.3) -> (51.9, 9.8)
  line L617 (47.4, 16.3) -> (46.7, 16.3)
  line L618 (39.1325, 55.32) -> (39.7675, 55.32)
  line L619 (47.4, 9.8) -> (46.7, 9.8)
  arc A79 (47.5, 15.3) -> (46.75, 15.25) centre (47.1467, 14.9498) ccw
  line L620 (26.115, 26.8238) -> (26.75, 26.8238)
  line L621 (51.2, 9.8) -> (51.2, 9.3)
  arc A80 (51.85, 15.25) -> (51.05, 15.25) centre (51.45, 14.95) ccw
  line L622 (28.02, 26.8238) -> (28.655, 26.8238)
  line L623 (39.1325, 55.32) -> (39.1325, 54.685)
  line L624 (36.9894, 55.32) -> (37.2275, 55.32)
  line L625 (46.7, 15.8) -> (47.4, 15.8)
  line L626 (28.02, 27.4588) -> (28.655, 27.4588)
  line L627 (28.8138, 33.57) -> (29.0519, 33.57)
  line L628 (28.8138, 32.935) -> (28.8138, 33.57)
  line L629 (39.7675, 55.32) -> (40.0056, 55.32)
  line L630 (37.8625, 54.685) -> (37.8625, 55.32)
  line L631 (27.7025, 28.7288) -> (28.02, 28.7288)
  line L632 (46.3, 10) -> (46.3, 10.05)
  line L633 (46.7, 9.3) -> (47.4, 9.3)
  line L634 (51.9, 15.8) -> (51.9, 16.3)
  line L635 (37.2275, 54.685) -> (37.8625, 54.685)
  line L636 (26.115, 27.4588) -> (26.115, 26.8238)
  line L637 (38.1006, 55.32) -> (37.8625, 55.32)
  line L638 (47.4, 9.3) -> (47.4, 9.8)
  line L639 (47.85, 9.8) -> (46.5, 9.8)
  line L640 (27.7025, 27.4588) -> (28.02, 27.4588)
  arc A81 (46.5, 15.8) -> (46.3, 15.6) centre (46.5, 15.6) ccw
  line L641 (28.655, 26.8238) -> (28.655, 27.4588)
  line L642 (38.18, 56.59) -> (38.815, 56.59)
  line L643 (51.2, 9.3) -> (51.9, 9.3)
  line L644 (52.3, 10.05) -> (52.3, 10)
  line L645 (51.9, 16.3) -> (51.2, 16.3)
  line L646 (27.8613, 33.57) -> (28.1788, 33.57)
  line L647 (51.2, 15.8) -> (51.9, 15.8)
  line L648 (47.4, 15.8) -> (47.4, 16.3)
  arc A82 (52.3, 15.6) -> (52.1, 15.8) centre (52.1, 15.6) ccw
  line L649 (37.2275, 55.32) -> (37.8625, 55.32)
  line L650 (38.18, 56.59) -> (37.8625, 56.59)
  line L651 (26.2737, 33.57) -> (26.2737, 32.935)
  line L652 (50.7, 15.8) -> (52.1, 15.8)
  line L653 (28.1788, 33.57) -> (28.1788, 32.935)
  line L654 (46.7, 9.8) -> (46.7, 9.3)
  line L655 (51.9, 9.8) -> (51.2, 9.8)
  line L656 (51.2, 16.3) -> (51.2, 15.8)
  arc A83 (46.8, 10.3) -> (47.55, 10.35) centre (47.1533, 10.6502) ccw
  line L657 (52.1, 9.8) -> (50.75, 9.8)
  arc A84 (52.1, 9.8) -> (52.3, 10) centre (52.1, 10) ccw
  arc A85 (51.1, 10.3) -> (51.85, 10.35) centre (51.4533, 10.6502) ccw
  line L658 (46.7, 16.3) -> (46.7, 15.8)
  line L659 (12.1915, 32.5398) -> (12.1915, 33.5558)
  line L660 (34.6869, 17.7006) -> (34.6869, 17.0656)
  line L661 (32.7819, 18.6531) -> (32.1469, 18.6531)
  line L662 (34.6869, 17.7006) -> (34.0519, 17.7006)
  line L663 (10.566, 33.5558) -> (10.566, 32.5398)
  line L664 (15.646, 28.6028) -> (15.646, 27.5868)
  line L665 (32.1469, 18.0181) -> (32.7819, 18.0181)
  line L666 (32.1469, 16.7481) -> (32.1469, 16.1131)
  line L667 (10.9216, 33.5558) -> (10.566, 33.5558)
  line L668 (13.4616, 28.6028) -> (13.106, 28.6028)
  line L669 (13.106, 33.5558) -> (13.106, 32.5398)
  line L670 (13.4616, 32.5398) -> (13.4616, 33.5558)
  line L671 (9.296, 27.5868) -> (9.6516, 27.5868)
  line L672 (9.6516, 27.5868) -> (9.6516, 28.6028)
  line L673 (15.646, 32.5398) -> (16.0016, 32.5398)
  line L674 (16.0016, 33.5558) -> (15.646, 33.5558)
  line L675 (10.9216, 27.5868) -> (10.9216, 28.6028)
  line L676 (9.296, 33.5558) -> (9.296, 32.5398)
  line L677 (10.566, 32.5398) -> (10.9216, 32.5398)
  line L678 (12.1915, 33.5558) -> (11.8359, 33.5558)
  line L679 (16.0016, 28.6028) -> (15.646, 28.6028)
  line L680 (14.7316, 27.5868) -> (14.7316, 28.6028)
  line L681 (14.376, 32.5398) -> (14.7316, 32.5398)
  line L682 (13.4616, 27.5868) -> (13.4616, 28.6028)
  line L683 (11.8359, 28.6028) -> (11.8359, 27.5868)
  line L684 (11.8359, 27.5868) -> (12.1915, 27.5868)
  line L685 (12.1915, 27.5868) -> (12.1915, 28.6028)
  line L686 (13.106, 28.6028) -> (13.106, 27.5868)
  line L687 (13.106, 32.5398) -> (13.4616, 32.5398)
  line L688 (14.7316, 32.5398) -> (14.7316, 33.5558)
  line L689 (14.376, 33.5558) -> (14.376, 32.5398)
  line L690 (16.0016, 27.5868) -> (16.0016, 28.6028)
  line L691 (14.376, 27.5868) -> (14.7316, 27.5868)
  line L692 (13.4616, 33.5558) -> (13.106, 33.5558)
  line L693 (15.646, 27.5868) -> (16.0016, 27.5868)
  line L694 (15.646, 33.5558) -> (15.646, 32.5398)
  line L695 (14.376, 28.6028) -> (14.376, 27.5868)
  line L696 (9.6516, 32.5398) -> (9.6516, 33.5558)
  line L697 (10.9216, 32.5398) -> (10.9216, 33.5558)
  line L698 (11.8359, 32.5398) -> (12.1915, 32.5398)
  line L699 (11.8359, 33.5558) -> (11.8359, 32.5398)
  line L700 (10.9216, 28.6028) -> (10.566, 28.6028)
  line L701 (14.7316, 33.5558) -> (14.376, 33.5558)
  line L702 (14.7316, 28.6028) -> (14.376, 28.6028)
  line L703 (9.296, 32.5398) -> (9.6516, 32.5398)
  line L704 (10.566, 27.5868) -> (10.9216, 27.5868)
  line L705 (12.1915, 28.6028) -> (11.8359, 28.6028)
  line L706 (13.106, 27.5868) -> (13.4616, 27.5868)
  line L707 (10.566, 28.6028) -> (10.566, 27.5868)
  line L708 (16.0016, 32.5398) -> (16.0016, 33.5558)
  line L709 (9.6516, 33.5558) -> (9.296, 33.5558)
  arc A86 (33.11, 3) -> (32.11, 3) centre (32.61, 3) ccw
  line L710 (33.11, 3) -> (33.11, 2)
  line L711 (48.95, 3) -> (48.95, 2)
  line L712 (32.7819, 18.8912) -> (32.7819, 18.6531)
  line L713 (10.2993, 28.6663) -> (11.1883, 28.6663)
  line L714 (32.7819, 17.78) -> (32.7819, 18.0181)
  line L715 (32.7819, 16.7481) -> (32.7819, 16.1131)
  arc A87 (37.07, 3) -> (36.07, 3) centre (36.57, 3) ccw
  line L716 (11.5693, 32.4763) -> (12.4583, 32.4763)
  line L717 (36.07, 3) -> (36.07, 2)
  line L718 (47.45, 0.1) -> (47.45, 4)
  line L719 (43.49, 0.1) -> (43.49, 4)
  line L720 (40.03, 3) -> (40.03, 2)
  line L721 (9.0293, 28.6663) -> (9.9183, 28.6663)
  arc A88 (37.57, 4) -> (35.57, 4) centre (36.57, 4) ccw
  arc A89 (36.07, 2) -> (37.07, 2) centre (36.57, 2) ccw
  line L722 (12.8392, 32.4763) -> (13.7283, 32.4763)
  line L723 (8.3816, 32.5398) -> (8.3816, 33.5558)
  arc A90 (41.53, 4) -> (39.53, 4) centre (40.53, 4) ccw
  line L724 (34.0519, 17.7006) -> (34.0519, 18.0181)
  arc A91 (43.99, 2) -> (44.99, 2) centre (44.49, 2) ccw
  arc A92 (44.99, 3) -> (43.99, 3) centre (44.49, 3) ccw
  line L725 (35.57, 0.1) -> (35.57, 4)
  line L726 (43.99, 3) -> (43.99, 2)
  line L727 (8.3816, 28.6028) -> (8.026, 28.6028)
  line L728 (45.49, 0.1) -> (45.49, 4)
  arc A93 (33.61, 4) -> (31.61, 4) centre (32.61, 4) ccw
  arc A94 (40.03, 2) -> (41.03, 2) centre (40.53, 2) ccw
  line L729 (39.53, 0.1) -> (39.53, 4)
  line L730 (32.7819, 16.1131) -> (32.7819, 15.875)
  arc A95 (48.95, 3) -> (47.95, 3) centre (48.45, 3) ccw
  line L731 (32.1469, 18.6531) -> (32.1469, 18.0181)
  line L732 (10.2993, 32.4763) -> (11.1883, 32.4763)
  line L733 (9.0293, 32.4763) -> (9.9183, 32.4763)
  arc A96 (41.03, 3) -> (40.03, 3) centre (40.53, 3) ccw
  line L734 (32.7819, 16.7481) -> (32.1469, 16.7481)
  line L735 (32.1469, 16.1131) -> (32.7819, 16.1131)
  line L736 (34.6869, 17.0656) -> (34.0519, 17.0656)
  line L737 (8.026, 33.5558) -> (8.026, 32.5398)
  arc A97 (49.45, 4) -> (47.45, 4) centre (48.45, 4) ccw
  line L738 (47.95, 3) -> (47.95, 2)
  line L739 (44.99, 3) -> (44.99, 2)
  line L740 (11.5693, 28.6663) -> (12.4583, 28.6663)
  line L741 (9.296, 28.6028) -> (9.296, 27.5868)
  line L742 (15.3793, 32.4763) -> (16.2683, 32.4763)
  line L743 (32.7819, 17.0656) -> (32.7819, 16.7481)
  line L744 (8.026, 32.5398) -> (8.3816, 32.5398)
  line L745 (32.7819, 18.6531) -> (32.7819, 18.0181)
  line L746 (14.1093, 28.6663) -> (14.9983, 28.6663)
  line L747 (34.0519, 17.7006) -> (34.0519, 17.0656)
  line L748 (12.8392, 28.6663) -> (13.7283, 28.6663)
  line L749 (34.0519, 17.0656) -> (34.0519, 16.7481)
  line L750 (8.3816, 33.5558) -> (8.026, 33.5558)
  line L751 (8.6483, 32.4763) -> (7.7593, 32.4763)
  arc A98 (47.95, 2) -> (48.95, 2) centre (48.45, 2) ccw
  line L752 (33.61, 0.1) -> (33.61, 4)
  line L753 (9.6516, 28.6028) -> (9.296, 28.6028)
  line L754 (31.61, 0.1) -> (31.61, 4)
  line L755 (8.026, 27.5868) -> (8.3816, 27.5868)
  line L756 (15.3793, 28.6663) -> (16.2683, 28.6663)
  line L757 (14.1093, 32.4763) -> (14.9983, 32.4763)
  line L758 (8.6483, 28.6663) -> (7.7593, 28.6663)
  line L759 (37.07, 3) -> (37.07, 2)
  line L760 (17.77, 0.1) -> (17.77, 4)
  line L761 (8.026, 28.6028) -> (8.026, 27.5868)
  line L762 (13.81, 0.1) -> (13.81, 4)
  arc A99 (21.23, 3) -> (20.23, 3) centre (20.73, 3) ccw
  line L763 (11.81, 0.1) -> (11.81, 4)
  line L764 (13.31, 3) -> (13.31, 2)
  line L765 (16.27, 3) -> (16.27, 2)
  line L766 (12.31, 3) -> (12.31, 2)
  arc A100 (25.19, 3) -> (24.19, 3) centre (24.69, 3) ccw
  line L767 (23.69, 0.1) -> (23.69, 4)
  line L768 (32.11, 3) -> (32.11, 2)
  arc A101 (29.15, 3) -> (28.15, 3) centre (28.65, 3) ccw
  line L769 (25.69, 0.1) -> (25.69, 4)
  line L770 (21.73, 0.1) -> (21.73, 4)
  line L771 (19.73, 0.1) -> (19.73, 4)
  line L772 (17.27, 3) -> (17.27, 2)
  arc A102 (29.65, 4) -> (27.65, 4) centre (28.65, 4) ccw
  arc A103 (12.31, 2) -> (13.31, 2) centre (12.81, 2) ccw
  line L773 (28.15, 3) -> (28.15, 2)
  line L774 (27.65, 0.1) -> (27.65, 4)
  line L775 (41.03, 3) -> (41.03, 2)
  arc A104 (17.27, 3) -> (16.27, 3) centre (16.77, 3) ccw
  arc A105 (45.49, 4) -> (43.49, 4) centre (44.49, 4) ccw
  arc A106 (21.73, 4) -> (19.73, 4) centre (20.73, 4) ccw
  arc A107 (25.69, 4) -> (23.69, 4) centre (24.69, 4) ccw
  arc A108 (13.31, 3) -> (12.31, 3) centre (12.81, 3) ccw
  line L776 (24.19, 3) -> (24.19, 2)
  arc A109 (28.15, 2) -> (29.15, 2) centre (28.65, 2) ccw
  line L777 (41.53, 0.1) -> (41.53, 4)
  arc A110 (8.35, 2) -> (9.35, 2) centre (8.85, 2) ccw
  line L778 (8.3816, 27.5868) -> (8.3816, 28.6028)
  line L779 (21.23, 3) -> (21.23, 2)
  arc A111 (13.81, 4) -> (11.81, 4) centre (12.81, 4) ccw
  line L780 (29.65, 0.1) -> (29.65, 4)
  line L781 (3.89, 0.1) -> (3.89, 4)
  arc A112 (16.27, 2) -> (17.27, 2) centre (16.77, 2) ccw
  line L782 (25.19, 3) -> (25.19, 2)
  arc A113 (32.11, 2) -> (33.11, 2) centre (32.61, 2) ccw
  line L783 (5.89, 0.1) -> (5.89, 4)
  arc A114 (20.23, 2) -> (21.23, 2) centre (20.73, 2) ccw
  line L784 (20.23, 3) -> (20.23, 2)
  line L785 (29.15, 3) -> (29.15, 2)
  arc A115 (17.77, 4) -> (15.77, 4) centre (16.77, 4) ccw
  arc A116 (24.19, 2) -> (25.19, 2) centre (24.69, 2) ccw
  line L786 (15.77, 0.1) -> (15.77, 4)
  line L787 (37.57, 0.1) -> (37.57, 4)
  line L788 (49.45, 0.1) -> (49.45, 4)
  circle A117 centre (12, 54.7) radius 1.5
  line L789 (23.1934, 17.9546) -> (22.6854, 17.9546)
  line L790 (9.35, 3) -> (9.35, 2)
  line L791 (27.7654, 17.4466) -> (28.2734, 17.4466)
  line L792 (15.5734, 17.4466) -> (15.5734, 17.9546)
  line L793 (11.2, 56.2) -> (12.8, 56.2)
  arc A118 (5.89, 4) -> (3.89, 4) centre (4.89, 4) ccw
  line L794 (5.39, 3) -> (5.39, 2)
  line L795 (12.3619, 55.7558) -> (12.3619, 55.5469)
  line L796 (12.1531, 55.3381) -> (11.6309, 55.3381)
  line L797 (25.7334, 17.9546) -> (25.2254, 17.9546)
  line L798 (12.127, 53.8863) -> (12.127, 53.4164)
  line L799 (11.4221, 55.5469) -> (11.4221, 55.7558)
  arc A119 (9.85, 4) -> (7.85, 4) centre (8.85, 4) ccw
  line L800 (9.85, 0.1) -> (9.85, 4)
  line L801 (7.85, 0.1) -> (7.85, 4)
  line L802 (8.35, 3) -> (8.35, 2)
  line L803 (18.1134, 17.4466) -> (18.1134, 17.9546)
  line L804 (11.4221, 53.6514) -> (12.3619, 53.9646)
  arc A120 (12.1531, 55.3381) -> (12.3619, 55.5469) centre (12.1531, 55.5469) ccw
  arc A121 (5.39, 3) -> (4.39, 3) centre (4.89, 3) ccw
  line L805 (25.2254, 17.9546) -> (25.2254, 17.4466)
  line L806 (30.3054, 17.9546) -> (30.3054, 17.4466)
  line L807 (13.0334, 17.4466) -> (13.0334, 17.9546)
  line L808 (25.7334, 17.4466) -> (25.7334, 17.9546)
  arc A122 (11.2, 53.2) -> (12.8, 53.2) centre (12, 54.7) ccw
  line L809 (20.1454, 17.4466) -> (20.6534, 17.4466)
  line L810 (12.3619, 53.3381) -> (11.4221, 53.6514)
  line L811 (22.6854, 17.4466) -> (23.1934, 17.4466)
  line L812 (13.0334, 17.9546) -> (12.5254, 17.9546)
  arc A123 (11.422, 55.547) -> (11.6309, 55.3381) centre (11.6309, 55.547) ccw
  line L813 (20.6534, 17.4466) -> (20.6534, 17.9546)
  line L814 (30.3054, 17.4466) -> (30.8134, 17.4466)
  line L815 (30.8134, 17.4466) -> (30.8134, 17.9546)
  arc A124 (9.35, 3) -> (8.35, 3) centre (8.85, 3) ccw
  line L816 (4.39, 3) -> (4.39, 2)
  line L817 (15.0654, 17.9546) -> (15.0654, 17.4466)
  line L818 (22.6854, 17.9546) -> (22.6854, 17.4466)
  line L819 (17.6054, 17.4466) -> (18.1134, 17.4466)
  arc A125 (4.39, 2) -> (5.39, 2) centre (4.89, 2) ccw
  line L820 (20.1454, 17.9546) -> (20.1454, 17.4466)
  line L821 (25.2254, 17.4466) -> (25.7334, 17.4466)
  line L822 (12.5254, 17.9546) -> (12.5254, 17.4466)
  line L823 (30.8134, 17.9546) -> (30.3054, 17.9546)
  line L824 (15.0654, 17.4466) -> (15.5734, 17.4466)
  arc A126 (7.2, 53.2) -> (8.8, 53.2) centre (8, 54.7) ccw
  circle A127 centre (24, 54.7) radius 1.5
  line L825 (23.4221, 55.5469) -> (23.4221, 55.7558)
  arc A128 (19.422, 55.547) -> (19.6309, 55.3381) centre (19.6309, 55.547) ccw
  line L826 (8.3619, 53.3381) -> (7.4221, 53.6514)
  line L827 (20.3619, 55.7558) -> (20.3619, 55.5469)
  line L828 (28.2734, 17.4466) -> (28.2734, 17.9546)
  line L829 (16.3619, 53.3381) -> (15.4221, 53.6514)
  line L830 (16.127, 53.8863) -> (16.127, 53.4164)
  line L831 (20.1531, 55.3381) -> (19.6309, 55.3381)
  arc A129 (8.1531, 55.3381) -> (8.3619, 55.5469) centre (8.1531, 55.5469) ccw
  arc A130 (23.2, 53.2) -> (24.8, 53.2) centre (24, 54.7) ccw
  line L832 (15.4221, 53.6514) -> (16.3619, 53.9646)
  line L833 (15.2, 56.2) -> (16.8, 56.2)
  arc A131 (7.422, 55.547) -> (7.6309, 55.3381) centre (7.6309, 55.547) ccw
  line L834 (24.1531, 55.3381) -> (23.6309, 55.3381)
  line L835 (7.2, 56.2) -> (8.8, 56.2)
  arc A132 (23.422, 55.547) -> (23.6309, 55.3381) centre (23.6309, 55.547) ccw
  line L836 (28.3619, 55.7558) -> (28.3619, 55.5469)
  arc A133 (27.422, 55.547) -> (27.6309, 55.3381) centre (27.6309, 55.547) ccw
  circle A134 centre (8, 54.7) radius 1.5
  arc A135 (24.1531, 55.3381) -> (24.3619, 55.5469) centre (24.1531, 55.5469) ccw
  line L837 (18.1134, 17.9546) -> (17.6054, 17.9546)
  line L838 (28.3619, 53.3381) -> (27.4221, 53.6514)